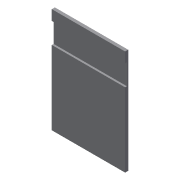
# Autodesk Inventor part: 00_chip_01_old
Saved by Autodesk Inventor 2019 (Build 230136000, 136)
## iProperties
Created: 2020-05-10
Part Number: 00_chip_01_old
Material: Generic
Document SubType Name: Modeling
Designer: diederichbenedict
Density: 1 g/cm^3
Appearance: Default
Author: diederichbenedict
Autodesk Inventor part; units mm, degrees
ref_plane "YZ Plane" through (0, 0, 0) normal (1, 0, 0) x (0, 1, 0)
ref_plane "XZ Plane" through (0, 0, 0) normal (0, 1, 0) x (-1, 0, 0)
ref_plane "XY Plane" through (0, 0, 0) normal (0, 0, 1) x (1, 0, 0)
sketch "Sketch1" plane through (0, 0, 0) normal (0, 0, 1) x (1, 0, 0)
  line L0 (0, 0) -> (23.76, 0)
  line L1 (23.76, 0) -> (23.76, 27)
  line L2 (23.76, 27) -> (0, 27)
  line L3 (0, 27) -> (0, 0)
  dimension "d0" = 23.76
  dimension "d1" = 27
  constraints: 8 end point, 2 parallel, 1 horizontal, 1 perpendicular
  measures "d0" distance of L2.end L1.end
  measures "d1" distance of L1.end L0.end
extrude "Extrusion1" add sketch "Sketch1" along normal blind 1
sketch "Sketch2" plane through (0, 0, 1) normal (0, 0, 1) x (1, 0, 0)
  line L0 (0, 0) -> (23.76, 0) projected
  line L1 (23.76, 0) -> (23.76, 27) projected
  line L2 (23.76, 27) -> (0, 27) projected
  line L3 (0, 27) -> (0, 0) projected
  line L4 (23.76, 0) -> (23.76, 27) projected
  line L5 (0, 23.7) -> (23.76, 23.7)
  line L6 (23.76, 23.7) -> (23.76, 16.95)
  line L7 (23.76, 16.95) -> (0, 16.95)
  line L8 (0, 16.95) -> (0, 23.7)
  line L9 (3.4, 24.9714) -> (18.51, 24.9714)
  line L10 (18.51, 24.9714) -> (18.51, 13.5)
  line L11 (18.51, 13.5) -> (3.4, 13.5)
  line L12 (3.4, 13.5) -> (3.4, 24.9714)
  dimension "d4" = 6.75
  dimension "d5" = 3.3
  dimension "d9" = 3.4
  dimension "d10" = 5.25
  constraints: 16 end point, 4 parallel, 2 horizontal, 2 perpendicular, 2 point on line
  measures "d4" distance of L5.end L6.end
  measures "d5" distance between parallel lines of L5 L2
  measures "d9" distance between parallel lines of L12 L3
  measures "d10" distance between parallel lines of L1 L10
extrude "Extrusion2" cut sketch "Sketch2" against normal blind 0.6 contours L3 L5 L12 L7 | L7 L10 L5 L1 | L12 L5 L10 L7 | L7 L10 L11 L12 | L12 L9 L10 L5
sketch "Sketch3" plane through (23.76, 0, 0) normal (1, 0, 0) x (0, 0, -1)
  line L0 (-0.4, 16.95) -> (-1, 16.95) projected
  line L1 (-1, 0) -> (-1, 16.95) projected
  line L2 (0, 0) -> (-1, 0) projected
  line L3 (0, 0) -> (0, 27) projected
  line L4 (0, 27) -> (-1, 27) projected
  line L5 (-1, 23.7) -> (-1, 27) projected
  line L6 (-1, 23.7) -> (-0.4, 23.7) projected
  line L7 (-0.4, 23.7) -> (-0.4, 16.95) projected
  circle A0 centre (-0.5521, 23.2257) radius 0.1521
  line L8 (-0.4, 23.7) -> (-0.4, 16.95) projected
  point P0 (0, 0)
  constraints: 1 centre point, 1 tangent
extrude "Extrusion3" add sketch "Sketch3" against normal up to surface (20.36 mm away) contours A0
pattern_linear "Rectangular Pattern1" count 24 spacing 0.27 along (0, -1, 0) of "Extrusion3"
body "Solid1"
